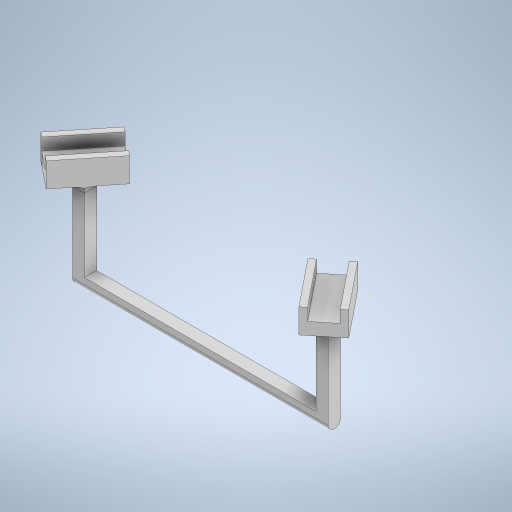
# Autodesk Inventor part: landingclasp
Saved by Autodesk Inventor 2023 (Build 270158000, 158)
## iProperties
Created: 2022-11-30
Part Number: landingclasp
Material: Generic
Document SubType Name: Modeling
Designer: user
Density: 1 g/cm^3
Appearance: Default
Author: user
## iProperties of the stored document landing_3DPrint.ipt
Created: 2022-11-30
Part Number: landing_3DPrint
Material: Generic
Document SubType Name: Modeling
Designer: user
Density: 1 g/cm^3
Appearance: Default
Author: user
Autodesk Inventor part; units mm, degrees
ref_plane "YZ Plane" through (0, 0, 0) normal (1, 0, 0) x (0, 1, 0)
ref_plane "XZ Plane" through (0, 0, 0) normal (0, 1, 0) x (-1, 0, 0)
ref_plane "XY Plane" through (0, 0, 0) normal (0, 0, 1) x (1, 0, 0)
sketch "Sketch1" plane through (0, 0, 0) normal (0, 0, 1) x (1, 0, 0)
  line L0 (0, 0) -> (133.35, 0)
  line L1 (133.35, 0) -> (133.35, 50.8)
  line L2 (0, 50.8) -> (0, 0)
  line L3 (0, 50.8) -> (6.35, 50.8)
  line L4 (6.35, 50.8) -> (6.35, 6.35)
  line L5 (6.35, 6.35) -> (127, 6.35)
  line L6 (127, 6.35) -> (127, 50.8)
  line L7 (127, 50.8) -> (133.35, 50.8)
  dimension "d1" = 50.8
  dimension "d2" = 6.35
  dimension "d3" = 44.45
  dimension "d4" = 120.65
  dimension "d5" = 133.35
  constraints: 16 end point, 3 perpendicular, 2 horizontal, 1 parallel
  measures "d1" distance of L0.end L1.end
  measures "d2" distance of L2.start L3.end
  measures "d3" distance of L3.end L4.end
  measures "d4" distance of L4.end L5.end
  measures "d5" distance of L0.start L0.end
extrude "Extrusion1" add sketch "Sketch1" along normal blind 6.35
fillet "Fillet1" radius 3.175 2 edges at (66.675, 0, 6.35) (66.675, 0, 0)
sketch "Sketch2" plane through (0, 50.8, 0) normal (0, 1, 0) x (1, 0, 0)
  line L0 (6.35, -6.35) -> (16.515747, 6.26204)
  line L1 (-2.903527, -17.830303) -> (6.35, -6.35)
  line L2 (16.515747, 6.26204) -> (9.563953, 11.86543)
  line L3 (9.563953, 11.86543) -> (-9.855321, -12.226913)
  line L4 (-9.855321, -12.226913) -> (-2.903527, -17.830303)
  line L5 (127, 0) -> (127, -6.35)
  line L6 (127, -6.35) -> (143.198942, -6.35) construction
  line L7 (116.834265, 6.26204) -> (123.786067, 11.86543)
  line L8 (123.786067, 11.86543) -> (143.205318, -12.226913)
  line L9 (143.205318, -12.226913) -> (136.253516, -17.830303)
  line L10 (133.35, -6.35) -> (127, -6.35)
  line L11 (116.834265, 6.26204) -> (136.253516, -17.830303)
  point P0 (0, 0)
  constraints: 20 end point, 4 perpendicular, 1 collinear, 1 horizontal
extrude "Extrusion2" add sketch "Sketch2" along normal blind 6.35
sketch "Sketch4" plane through (16.515747, 50.8, -6.26204) normal (0.7785715, 0, 0.6275559) x (0.6275559, 0, -0.7785715)
  point P0 (-15.240001, -50.8)
sketch "Sketch5" plane through (16.515747, 50.8, -6.26204) normal (0.7785715, 0, 0.6275559) x (0.6275559, 0, -0.7785715)
  point P0 (-15.240001, -50.8)
sketch "Sketch6" plane through (16.515747, 50.8, -6.26204) normal (0.7785715, 0, 0.6275559) x (0.6275559, 0, -0.7785715)
  line L0 (-30.944292, 6.35) -> (0, 6.35)
  line L1 (-30.944292, 0) -> (-30.944292, 6.35)
  line L2 (-30.944292, 6.35) -> (-30.944292, 0)
  line L3 (0, 0) -> (0, 6.35)
  line L4 (-30.944292, 0) -> (0, 0)
  line L5 (0, 0) -> (0, 6.35)
  line L6 (0, 6.35) -> (-30.944292, 6.35)
  point P0 (-15.240001, -50.8)
  constraints: 8 end point, 2 collinear, 2 perpendicular
extrude "Extrusion3" add sketch "Sketch6" along normal blind 1.5875
sketch "Sketch7" plane through (-9.855321, 50.8, 12.226913) normal (-0.7785715, 0, -0.6275559) x (-0.6275559, 0, 0.7785715)
  line L0 (-30.944292, 6.35) -> (0, 6.35)
  line L1 (0, 0) -> (-30.944292, 0)
  line L2 (-30.944292, 6.35) -> (-30.944292, 0)
  line L3 (-30.944292, 0) -> (0, 0)
  line L4 (0, 6.35) -> (0, 0)
  line L5 (0, 0) -> (0, 6.35)
  line L6 (0, 6.35) -> (-30.944292, 6.35)
  point P0 (-15.704291, -50.8)
  constraints: 8 end point, 2 collinear, 1 perpendicular, 1 vertical
extrude "Extrusion4" add sketch "Sketch7" along normal blind 1.5875
sketch "Sketch8" plane through (136.253516, 50.8, 17.830303) normal (-0.7785718, 0, 0.6275555) x (0.6275555, 0, 0.7785718)
  line L0 (-30.944277, 6.35) -> (0, 6.35)
  line L1 (0, 0) -> (0, 6.35)
  line L2 (-30.944277, 6.35) -> (0, 6.35)
  line L3 (0, 6.35) -> (0, 0)
  line L4 (0, 0) -> (-30.944277, 0)
  line L5 (-30.944277, 0) -> (-30.944277, 6.35)
  line L6 (-30.944277, 0) -> (-30.944277, 6.35)
  point P0 (-99.388813, -50.8)
  constraints: 8 end point, 3 perpendicular, 1 collinear
extrude "Extrusion5" add sketch "Sketch8" along normal blind 1.5875
sketch "Sketch9" plane through (123.786067, 50.8, -11.86543) normal (0.7785718, 0, -0.6275555) x (-0.6275555, 0, -0.7785718)
  line L0 (-30.944277, 6.35) -> (0, 6.35)
  line L1 (-30.944277, 6.35) -> (0, 6.35)
  line L2 (0, 0) -> (-30.944277, 0)
  line L3 (0, 6.35) -> (0, 0)
  line L4 (0, 0) -> (-30.944277, 0)
  line L5 (-30.944277, 0) -> (-30.944277, 6.35)
  point P0 (68.444536, -50.8)
  constraints: 8 end point, 2 collinear, 2 perpendicular
extrude "Extrusion6" add sketch "Sketch9" along normal blind 1.5875
sketch "Sketch10" plane through (125.02205, 50.8, -12.861674) normal (0.7785718, 0, -0.6275555) x (-0.6275555, 0, -0.7785718)
  point P0 (68.444536, -50.8)
sketch "Sketch11" plane through (125.02205, 50.8, -12.861674) normal (0.7785718, 0, -0.6275555) x (-0.6275555, 0, -0.7785718)
  line L0 (0, 0) -> (0, 6.35)
  line L1 (0, 0) -> (0, 12.7)
  line L2 (-30.944277, 6.35) -> (-30.944277, 0)
  line L3 (0, 0) -> (-30.944277, 0)
  line L4 (-30.944277, 0) -> (-30.944277, 12.7)
  line L5 (-30.944277, 12.7) -> (0, 12.7)
  point P0 (68.444536, -50.8)
  point P1 (0, 6.35)
  point P2 (-30.944277, 6.35)
  dimension "d40" = 12.7
  constraints: 8 end point, 2 perpendicular, 1 collinear, 1 horizontal
  measures "d40" distance of L0.start L1.end
extrude "Extrusion7" add sketch "Sketch11" along normal blind 3.175
sketch "Sketch12" plane through (135.017533, 50.8, 18.826547) normal (-0.7785718, 0, 0.6275555) x (0.6275555, 0, 0.7785718)
  line L0 (0, 12.7) -> (0, 0)
  line L1 (0, 0) -> (0, 12.7)
  line L2 (-30.944277, 12.7) -> (0, 12.7)
  line L3 (0, 12.7) -> (-30.944277, 12.7)
  line L4 (0, 0) -> (-30.944277, 0)
  line L5 (-30.944277, 12.7) -> (-30.944277, 0)
  line L6 (-30.944277, 0) -> (0, 0)
  point P0 (-99.388813, -50.8)
  constraints: 8 end point, 3 perpendicular, 1 collinear
extrude "Extrusion8" add sketch "Sketch12" along normal blind 3.175
sketch "Sketch13" plane through (-11.091303, 50.8, 11.230668) normal (-0.7785715, 0, -0.6275559) x (-0.6275559, 0, 0.7785715)
  line L0 (-30.944292, 0) -> (-30.944292, 6.35)
  line L1 (-30.944292, 0) -> (-30.944292, 12.7)
  line L2 (0, 6.35) -> (0, 0)
  line L3 (-30.944292, 0) -> (0, 0)
  line L4 (0, 0) -> (0, 12.7)
  line L5 (0, 12.7) -> (-30.944292, 12.7)
  point P0 (-15.704291, -50.8)
  point P1 (-30.944292, 6.35)
  dimension "d45" = 12.7
  constraints: 8 end point, 2 collinear, 1 horizontal, 1 perpendicular
  measures "d45" distance of L0.start L1.end
extrude "Extrusion9" add sketch "Sketch13" along normal blind 3.175
sketch "Sketch14" plane through (17.751729, 50.8, -5.265795) normal (0.7785715, 0, 0.6275559) x (0.6275559, 0, -0.7785715)
  line L0 (-30.944292, 0) -> (-30.944292, 6.35)
  line L1 (-30.944292, 0) -> (-30.944292, 12.7)
  line L2 (-30.944292, 12.7) -> (0, 12.7)
  line L3 (-30.944292, 12.7) -> (0, 12.7)
  line L4 (0, 0) -> (0, 6.35)
  line L5 (0, 12.7) -> (0, 0)
  line L6 (0, 0) -> (-30.944292, 0)
  point P0 (-15.240001, -50.8)
  point P1 (0, 6.35)
  point P2 (-30.944292, 12.7)
  point P3 (-30.944292, 6.35)
  dimension "d8" = 3.175
  constraints: 8 end point, 2 perpendicular, 1 collinear, 1 vertical
extrude "Extrusion10" add sketch "Sketch14" along normal blind 3.175
fillet "Fillet4" radius 6.35 8 edges at (133.35, 50.8, 3.175) (130.175, 50.8, 0) (127, 50.8, 3.175) (130.175, 50.8, 6.35) (6.35, 50.8, 3.175) (3.175, 50.8, 6.35) (0, 50.8, 3.175) (3.175, 50.8, 0)
body "Solid1"
